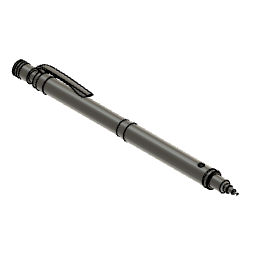
Uni Kuru toga roulette_ (Autodesk Fusion 360 design; units mm, degrees)
Autodesk Fusion 360 part; units mm, degrees
sketch "Sketch1" plane through (0, 0, 0) normal (0, 0, 1) x (1, 0, 0)
  line L0 (0, 0) -> (-2.5, 0)
  line L1 (-2.5, 0) -> (-2.5, 0.4)
  line L2 (-2.5, 0.4) -> (0, 0.4)
  line L3 (0, 0.4) -> (0, 0)
  line L4 (-2.5, 0) -> (-2.5, 1.3)
  line L5 (-2.5, 0) -> (-5.5, 0)
  line L6 (-5.5, 0) -> (-5.5, 1.5)
  line L7 (-2.5, 1.3) -> (-5.5, 1.5)
  line L8 (-5.5, 0) -> (-7.5, 0)
  line L9 (-7.5, 0) -> (-7.5, 2)
  line L10 (-7.5, 2) -> (-5.5, 2)
  line L11 (-5.5, 2) -> (-5.5, 0)
  line L12 (-7.5, 0) -> (-8.5, 0)
  line L13 (-8.5, 0) -> (-8.5, 3.25)
  line L14 (-7.5, 2) -> (-8.5, 3.25)
  line L15 (-8.5, 0) -> (-15.5, 0)
  line L16 (-15.5, 0) -> (-15.5, 3.5)
  line L17 (-8.5, 3.25) -> (-15.5, 3.5)
  line L18 (-15.5, 0) -> (-15.5, 4.5)
  line L19 (-15.5, 0) -> (-16, 0)
  line L20 (-16, 0) -> (-16, 4.75)
  line L21 (-15.5, 4.5) -> (-16, 4.75)
  line L22 (-16, 0) -> (-18, 0)
  line L23 (-18, 0) -> (-18, 4.75)
  line L24 (-18, 4.75) -> (-16, 4.75)
  line L25 (-18, 0) -> (-18.5, 0)
  line L26 (-18.5, 0) -> (-18.5, 4.75)
  line L27 (0, 0) -> (-71, 0)
  line L28 (-71, 0) -> (-71, 4.75)
  line L29 (-71, 4.75) -> (-18.5, 4.75)
  line L30 (-71, 0) -> (-76, 0)
  line L31 (-76, 0) -> (-76, 4.35)
  line L32 (-76, 4.35) -> (-71, 4.75)
  line L33 (-76, 0) -> (-125, 0)
  line L34 (-125, 0) -> (-125, 4.35)
  line L35 (-125, 4.35) -> (-76, 4.35)
  line L36 (-125, 0) -> (-129.5, 0)
  line L37 (-129.5, 0) -> (-129.5, 4.55)
  line L38 (-125, 0) -> (-125, 4.55)
  line L39 (-125, 4.55) -> (-129.5, 4.55)
  line L40 (-129.5, 0) -> (-132, 0)
  line L41 (-132, 0) -> (-132, 4.35)
  line L42 (-129.5, 0) -> (-129.5, 4.35)
  line L43 (-132, 4.35) -> (-129.5, 4.35)
  line L44 (-132, 0) -> (-136, 0)
  line L45 (-136, 0) -> (-136, 2.75)
  line L46 (-136, 2.75) -> (-132, 2.75)
  line L47 (-136, 0) -> (-141.5, 0)
  line L48 (-141.5, 0) -> (-141.5, 4)
  line L49 (-141.5, 4) -> (-136, 4)
  line L50 (-136, 4) -> (-136, 0)
  line L51 (-141.5, 0) -> (-144.5, 0)
  line L52 (-144.5, 0) -> (-144.5, 4)
  line L53 (-144.5, 4) -> (-145.5, 4)
  line L54 (-145.5, 4) -> (-145.5, 0)
  line L55 (-145.5, 0) -> (-144.5, 0)
  line L56 (-143, 0) -> (-143, 4.1)
  line L57 (-144.5, 4) -> (-143, 4.1)
  line L58 (-141.5, 4) -> (-143, 4.1)
  line L59 (-18.5, 4.75) -> (-18, 4.75)
  circle A0 centre (-18.25, 4.75) radius 0.25
  dimension "d1" = 2.5
  dimension "d2" = 0.4
  dimension "d3" = 1.3
  dimension "d4" = 3
  dimension "d5" = 1.5
  dimension "d6" = 2
  dimension "d7" = 2
  dimension "d8" = 1
  dimension "d9" = 3.25
  dimension "d10" = 7
  dimension "d11" = 3.5
  dimension "d12" = 4.5
  dimension "d13" = 0.5
  dimension "d14" = 4.75
  dimension "d15" = 2
  dimension "d16" = 0.5
  dimension "d17" = 4.75
  dimension "d18" = 71
  dimension "d19" = 4.75
  dimension "d20" = 4.35
  dimension "d21" = 49
  dimension "d22" = 4.35
  dimension "d23" = 4.5
  dimension "d24" = 4.55
  dimension "d25" = 4.55
  dimension "d26" = 2.5
  dimension "d27" = 4.35
  dimension "d28" = 4.35
  dimension "d29" = 4
  dimension "d30" = 2.75
  dimension "d31" = 5.5
  dimension "d32" = 4
  dimension "d33" = 3
  dimension "d34" = 1
  dimension "d35" = 4.1
  constraint horizontal L0
  constraint vertical L1
  constraint horizontal L2
  constraint vertical L3
  constraint coincident L0.start L3.end
  constraint perpendicular L2 L4
  constraint perpendicular L1 L5
  constraint perpendicular L5 L6
  constraint horizontal L8
  constraint vertical L9
  constraint horizontal L10
  constraint vertical L11
  constraint perpendicular L9 L12
  constraint perpendicular L12 L13
  constraint perpendicular L13 L15
  constraint perpendicular L15 L16
  constraint perpendicular L15 L18
  constraint perpendicular L18 L19
  constraint perpendicular L19 L20
  constraint perpendicular L20 L22
  constraint perpendicular L22 L23
  constraint perpendicular L20 L24
  constraint perpendicular L23 L25
  constraint perpendicular L25 L26
  constraint perpendicular L3 L27
  constraint perpendicular L27 L28
  constraint perpendicular L28 L30
  constraint perpendicular L27 L31
  constraint perpendicular L31 L33
  constraint perpendicular L33 L34
  constraint perpendicular L34 L36
  constraint perpendicular L36 L37
  constraint perpendicular L35 L38
  constraint perpendicular L37 L40
  constraint perpendicular L40 L41
  constraint perpendicular L36 L42
  constraint perpendicular L41 L44
  constraint perpendicular L44 L45
  constraint coincident L41 L46.end
  constraint perpendicular L41 L46
  constraint perpendicular L45 L47
  constraint perpendicular L47 L48
  constraint perpendicular L48 L49
  constraint perpendicular L48 L51
  constraint perpendicular L51 L52
  constraint perpendicular L52 L53
  constraint perpendicular L53 L54
  constraint perpendicular L52 L55
  constraint midpoint L51 L56.start
  constraint perpendicular L51 L56
  constraint midpoint L59 A0.centre
  constraint coincident L26.end A0
  measures "d1" distance of L0.start L0.end
  measures "d2" distance of L0.start L2.end
  measures "d3" distance of L0.end L4.end
  measures "d4" distance of L0.end L5.end
  measures "d5" distance of L5.end L6.end
  measures "d6" distance of L5.end L8.end
  measures "d7" distance of L5.end L10.end
  measures "d8" distance of L8.end L12.end
  measures "d9" distance of L12.end L13.end
  measures "d10" distance of L12.end L15.end
  measures "d11" distance of L15.end L16.end
  measures "d12" distance of L15.end L18.end
  measures "d13" distance of L15.end L19.end
  measures "d14" distance of L19.end L20.end
  measures "d15" distance of L19.end L22.end
  measures "d16" distance of L22.end L25.end
  measures "d17" distance of L25.end L26.end
  measures "d18" distance of L0.start L27.end
  measures "d19" distance of L27.end L28.end
  measures "d20" distance of L30.end L31.end
  measures "d21" distance of L30.end L33.end
  measures "d22" distance of L33.end L34.end
  measures "d23" distance of L33.end L36.end
  measures "d24" distance of L36.end L37.end
  measures "d25" distance of L33.end L38.end
  measures "d26" distance of L36.end L40.end
  measures "d27" distance of L40.end L41.end
  measures "d28" distance of L36.end L42.end
  measures "d29" distance of L40.end L44.end
  measures "d30" distance of L44.end L45.end
  measures "d31" distance of L44.end L47.end
  measures "d32" distance of L47.end L48.end
  measures "d33" distance of L47.end L51.end
  measures "d34" distance of L52.end L53.end
  measures "d35" distance of L56.start L56.end
revolve "Revolve1" add sketch "Sketch1" angle 360 about axis through (0, 0, 0) along (-1, 0, 0)
fillet "Fillet1" radius 0.1 1 edges at (-143, -1.4826, 3.8225)
fillet "Fillet2" radius 0.2 1 edges at (-132, -1.573, 4.0556)
move_body "Move1" bodies 1 to x (1, 0, 0) y (0, 1, 0) z (0, 0, 1) at (0, 0, 4.75)
sketch "Sketch2" plane through (0, 0, 0) normal (0, 0, 1) x (1, 0, 0)
  circle A0 centre (-24, -0.0016) radius 1.5
  line L0 (-18.5, -4.75) -> (-18.5, 4.75)
  dimension "d44" = 3
  dimension "d60" = 5.5
  measures "d44" diameter of A0
  measures "d60" distance of A0.centre L0
extrude "Extrude1" cut sketch "Sketch2" along normal blind 1
move_body "Move2" bodies 1 to x (1, 0, 0) y (0, -1, 0) z (0, 0, -1) at (0, 0, 9.5)
sketch "Sketch3" plane through (0, 0, 0) normal (0, 1, 0) x (1, 0, 0)
  spline S0 degree 5 poles (-131.8, -12.4) (-131.3149, -12.5617) (-130.1127, -12.8262) (-127.614, -13.0466) (-123.0836, -13.0362) (-116.0905, -12.6857) (-109.8433, -12.2397) (-104.9113, -11.8426) (-101.5208, -11.5519) (-99.8, -11.4) knots 0 0 0 0 0 0 0.2 0.4 0.6 0.8 1 1 1 1 1 1
  line L0 (-133, -12) -> (-130.6, -12.8)
  line L1 (-99.8, -0.4) -> (-103.8, -0.4)
  line L2 (-99.8, -0.4) -> (-110.8, -0.4)
  spline S1 degree 5 poles (-131.8, -12.4) (-132.224, -12.1577) (-132.9215, -11.7053) (-133.5163, -11.1231) (-133.531, -10.5133) (-132.686, -9.9356) (-131.5862, -9.5641) (-130.6013, -9.3196) (-129.8782, -9.1708) (-129.5, -9.1) knots 0 0 0 0 0 0 0.2 0.4 0.6 0.8 1 1 1 1 1 1
  line L3 (-131.1, -12.8) -> (-132.5, -12)
  spline S2 degree 5 poles (-99.8, -11.4) (-99.9437, -11.2107) (-100.238, -10.8494) (-100.7004, -10.3593) (-101.3594, -9.8115) (-102.2587, -9.3136) (-103.239, -9.0168) (-104.3052, -8.9328) (-105.4566, -9.0604) (-106.6871, -9.3841) (-107.9894, -9.8859) (-109.0834, -10.4165) (-109.9312, -10.8823) (-110.5084, -11.2225) (-110.8, -11.4) knots 0 0 0 0 0 0 0.1 0.2 0.3 0.4 0.5 0.6 0.7 0.8 0.9 1 1 1 1 1 1
  spline S3 degree 5 poles (-129.5, -9.3) (-129.819, -9.3818) (-130.4125, -9.5432) (-131.1691, -9.7786) (-131.9101, -10.0787) (-132.3942, -10.4306) (-132.4575, -10.7578) (-132.1469, -11.058) (-131.5494, -11.3271) (-130.7831, -11.5599) (-129.9736, -11.7484) (-129.2306, -11.8842) (-128.6356, -11.9512) (-128.1685, -11.9634) (-127.755, -11.9496) (-127.3052, -11.9384) (-126.7589, -11.9425) (-126.0816, -11.9615) (-125.2561, -11.9875) (-124.2763, -12.0098) (-123.1393, -12.0197) (-121.8441, -12.0109) (-120.3914, -11.979) (-118.783, -11.9211) (-117.0211, -11.8356) (-115.1082, -11.7215) (-113.4586, -11.6072) (-112.1551, -11.5086) (-111.2566, -11.4372) (-110.8, -11.4) knots 0 0 0 0 0 0 0.04 0.08 0.12 0.16 0.2 0.24 0.28 0.32 0.36 0.4 0.44 0.48 0.52 0.56 0.6 0.64 0.68 0.72 0.76 0.8 0.84 0.88 0.92 0.96 1 1 1 1 1 1
  line L4 (-132.2274, -11.3537) -> (-126.8, -12.3)
  line L5 (-129.5, -9.1) -> (-129.5, -9.3)
  point P0 (-103.8, -9)
  point P1 (-132.2875, -10.8754)
  point P2 (-129.5137, -11.8269)
  point P3 (-127.6973, -11.9489)
  point P4 (-125.0898, -11.9898)
  dimension "d51" = 11
  dimension "d52" = 4
  dimension "d53" = 11
  dimension "d54" = 11
  constraint midpoint S0.start L0
  constraint midpoint S0.start L3
  constraint midpoint P2 L4
  constraint vertical L5
  measures "d51" distance of L1.start S0.end
  measures "d52" distance of L1.start L1.end
  measures "d53" distance of L1.start L2.end
  measures "d54" distance of L2.end S2.end
revolve "Revolve2" add sketch "Sketch3" angle 36 about axis through (-125, 0, 4.75) along (-1, 0, 0)
equation "d20 = ( 8.7 / 2 ) * 1 mm"
equation "d24 = ( 9.1 / 2 ) * 1 mm"
equation "d30 = ( 5.5 / 2 ) * 1 mm"
equation "d59 = ( 360 / 10 ) * 1 deg"
equation "d60 = 4 mm + d44 / 2"
